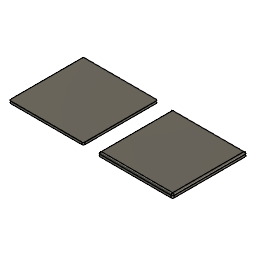
New Pressure Plate (Autodesk Fusion 360 design; units mm, degrees)
Autodesk Fusion 360 part; units mm, degrees
sketch "Sketch1" plane through (0, 0, 0) normal (0, 0, 1) x (1, 0, 0)
  line L0 (25, -25) -> (-25, -25)
  line L1 (-25, -25) -> (-25, 25)
  line L2 (-25, 25) -> (25, 25)
  line L3 (25, 25) -> (25, -25)
  line L4 (25, -25) -> (-25, 25) construction
  line L5 (-25, -25) -> (25, 25) construction
  line L6 (85, -25) -> (35, -25)
  line L7 (35, -25) -> (35, 25)
  line L8 (85, -25) -> (35, 25) construction
  line L9 (35, 25) -> (85, 25)
  line L10 (35, -25) -> (85, 25) construction
  line L11 (85, 25) -> (85, -25)
  point P0 (60, 0)
  point P1 (60, 0)
  dimension "d1" = 50
  dimension "d2" = 50
  dimension "d3" = 50
  dimension "d4" = 50
  constraint horizontal L0
  constraint perpendicular L0 L1
  constraint parallel L0 L2
  constraint parallel L1 L3
  constraint coincident L4 origin
  constraint coincident L5 origin
  constraint horizontal L6
  constraint perpendicular L6 L7
  constraint parallel L6 L9
  constraint parallel L7 L11
  constraint coincident P1 L8
  constraint coincident P1 L10
  constraint coincident P1 P0
  measures "d1" distance of L1.end L2.end
  measures "d2" distance of L0.end L1.end
  measures "d3" distance of L7.end L9.end
  measures "d4" distance of L6.end L7.end
extrude "Extrude1" add sketch "Sketch1" along normal blind 2 makes body 1 at (8.3333, -8.3333, 0) makes body 2 at (68.3333, -8.3333, 0)
fillet "Fillet1" radius 1 12 edges at (25, 25, 1) (25, -25, 1) (-25, -25, 1) (-25, 25, 1) (85, 25, 1) (60, 25, 2) (85, 0, 2) (35, -25, 1) (60, -25, 2) (85, -25, 1) (35, 0, 2) (35, 25, 1) on bodies 1 2
sketch "Sketch2" plane through (0, 0, 0) normal (0, 0, -1) x (1, 0, 0)
  arc A0 (-25, -24) -> (-24, -25) centre (-24, -24) ccw
  line L0 (-24, -25) -> (24, -25)
  arc A1 (24, -25) -> (25, -24) centre (24, -24) ccw
  line L1 (25, -24) -> (25, 24)
  arc A2 (25, 24) -> (24, 25) centre (24, 24) ccw
  line L2 (24, 25) -> (-24, 25)
  arc A3 (-24, 25) -> (-25, 24) centre (-24, 24) ccw
  line L3 (-25, 24) -> (-25, -24)
  line L4 (-24, -24) -> (24, -24)
  line L5 (24, -24) -> (24, 24)
  line L6 (24, 24) -> (-24, 24)
  line L7 (-24, 24) -> (-24, -24)
  dimension "d9" = -1
extrude "Extrude2" cut sketch "Sketch2" against normal blind 0.5 bodies 1
sketch "Sketch3" plane through (0, 0, 0) normal (0, 0, -1) x (1, 0, 0)
  arc A0 (36, 25) -> (35, 24) centre (36, 24) ccw
  line L0 (35, 24) -> (35, -24)
  arc A1 (35, -24) -> (36, -25) centre (36, -24) ccw
  line L1 (36, -25) -> (84, -25)
  arc A2 (84, -25) -> (85, -24) centre (84, -24) ccw
  line L2 (85, -24) -> (85, 24)
  arc A3 (85, 24) -> (84, 25) centre (84, 24) ccw
  line L3 (84, 25) -> (36, 25)
  line L4 (36, -24) -> (84, -24)
  line L5 (84, -24) -> (84, 24)
  line L6 (84, 24) -> (36, 24)
  line L7 (36, 24) -> (36, -24)
  dimension "d12" = -1
extrude "Extrude3" add sketch "Sketch3" along normal blind 0.5 bodies 2
sketch "Sketch4" plane through (0, 24, 0) normal (0, -1, 0) x (1, 0, 0)
  line L0 (84, 0) -> (36, 0)
  line L1 (36, 0) -> (36, -0.5)
  line L2 (36, -0.5) -> (84, -0.5)
  line L3 (84, -0.5) -> (84, 0)
  line L4 (84, -0.5) -> (60, -0.5)
  line L5 (60, -0.5) -> (61, -0.5)
  line L6 (61, -0.5) -> (61, 0)
  line L7 (61, 0) -> (60, 0)
  line L8 (60, 0) -> (60, -0.5)
  line L9 (60, -0.5) -> (59, -0.5)
  line L10 (59, -0.5) -> (59, 0)
  line L11 (59, 0) -> (60, 0)
  line L12 (60, 0) -> (60, -0.5)
  constraint coincident L2.end L3.start
  constraint midpoint L2 L4.end
  constraint horizontal L5
  constraint vertical L6
  constraint horizontal L7
  constraint vertical L8
  constraint coincident L0 L6.end
  constraint horizontal L9
  constraint vertical L10
  constraint horizontal L11
  constraint vertical L12
  constraint coincident L0 L10.end
extrude "Extrude4" cut sketch "Sketch4" against normal up to surface (1 mm away) contours L0 L2 L4 L5 L6 L7 L8 L12 | L0 L2 L8 L9 L10 L11 L12 bodies 2
